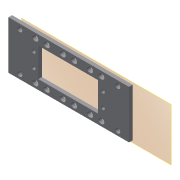
# Autodesk Inventor part: ExtendedServoMount
Saved by Autodesk Inventor 2018 (Build 220112000, 112)
## iProperties
Created: 2018-12-08
Part Number: ExtendedServoMount
Material: Generic
Document SubType Name: Modeling
Designer: ball
Density: 1 g/cm^3
Appearance: Default
Author: ball
Autodesk Inventor part; units mm, degrees
ref_plane "YZ Plane" through (0, 0, 0) normal (1, 0, 0) x (0, 1, 0)
ref_plane "XZ Plane" through (0, 0, 0) normal (0, 1, 0) x (-1, 0, 0)
ref_plane "XY Plane" through (0, 0, 0) normal (0, 0, 1) x (1, 0, 0)
ref_plane "Work Plane1" through (0, 0, 0) normal (0, 0, 1) x (1, 0, 0)
sketch "Sketch2" plane through (0, 0, 0) normal (0, 0, 1) x (1, 0, 0)
  arc A0 (-24.5984, 11.6916) -> (-24.5984, 15.2476) centre (-24.5984, 13.4696) ccw projected
  line L0 (-24.5984, 15.2476) -> (-25.3604, 15.2476) projected
  line L1 (-25.3604, 11.6916) -> (-24.5984, 11.6916) projected
  arc A1 (-25.3604, 15.2476) -> (-25.3604, 11.6916) centre (-25.3604, 13.4696) ccw projected
  arc A2 (-25.3604, 15.2476) -> (-25.3604, 11.6916) centre (-25.3604, 13.4696) ccw
  arc A3 (-24.5984, 11.6916) -> (-24.5984, 15.2476) centre (-24.5984, 13.4696) ccw
  line L2 (-27.1384, 13.4696) -> (-22.8204, 13.4696) construction
  line L3 (-25.3604, 11.6916) -> (-24.5984, 11.6916)
  line L4 (-24.5984, 15.2476) -> (-25.3604, 15.2476)
  arc A4 (-25.3604, 15.2476) -> (-25.3604, 11.6916) centre (-25.3604, 13.4696) ccw
  arc A5 (-24.5984, 11.6916) -> (-24.5984, 15.2476) centre (-24.5984, 13.4696) ccw
  arc A6 (-33.2496, 15.2476) -> (-33.2496, 11.6916) centre (-33.2496, 13.4696) ccw
  arc A7 (-32.4876, 11.6916) -> (-32.4876, 15.2476) centre (-32.4876, 13.4696) ccw
  arc A8 (-43.6499, 11.6916) -> (-43.6499, 15.2476) centre (-43.6499, 13.4696) ccw
  arc A9 (-44.4119, 15.2476) -> (-44.4119, 11.6916) centre (-44.4119, 13.4696) ccw projected
  arc A10 (-51.5391, 11.6916) -> (-51.5391, 15.2476) centre (-51.5391, 13.4696) ccw
  arc A11 (-52.3011, 15.2476) -> (-52.3011, 11.6916) centre (-52.3011, 13.4696) ccw projected
  line L5 (-46.1899, 13.4696) -> (-41.8719, 13.4696) construction
  line L6 (-44.4119, 11.6916) -> (-43.6499, 11.6916)
  line L7 (-43.6499, 15.2476) -> (-44.4119, 15.2476)
  arc A12 (-44.4119, 15.2476) -> (-44.4119, 11.6916) centre (-44.4119, 13.4696) ccw
  arc A13 (-43.6499, 11.6916) -> (-43.6499, 15.2476) centre (-43.6499, 13.4696) ccw
  line L8 (-54.0791, 13.4696) -> (-49.7611, 13.4696) construction
  line L9 (-52.3011, 11.6916) -> (-51.5391, 11.6916)
  line L10 (-51.5391, 15.2476) -> (-52.3011, 15.2476)
  arc A14 (-52.3011, 15.2476) -> (-52.3011, 11.6916) centre (-52.3011, 13.4696) ccw
  arc A15 (-51.5391, 11.6916) -> (-51.5391, 15.2476) centre (-51.5391, 13.4696) ccw
  line L11 (-35.0276, 13.4696) -> (-30.7096, 13.4696) construction
  line L12 (-33.2496, 11.6916) -> (-32.4876, 11.6916)
  line L13 (-32.4876, 15.2476) -> (-33.2496, 15.2476)
  arc A16 (-33.2496, 15.2476) -> (-33.2496, 11.6916) centre (-33.2496, 13.4696) ccw
  arc A17 (-32.4876, 11.6916) -> (-32.4876, 15.2476) centre (-32.4876, 13.4696) ccw
  line L14 (-65.2414, 13.4696) -> (-60.9234, 13.4696) construction
  line L15 (-63.4634, 11.6916) -> (-62.7014, 11.6916)
  line L16 (-62.7014, 15.2476) -> (-63.4634, 15.2476)
  arc A18 (-63.4634, 15.2476) -> (-63.4634, 11.6916) centre (-63.4634, 13.4696) ccw
  arc A19 (-62.7014, 11.6916) -> (-62.7014, 15.2476) centre (-62.7014, 13.4696) ccw
  line L17 (-73.1307, 13.4696) -> (-68.8127, 13.4696) construction
  line L18 (-71.3527, 11.6916) -> (-70.5907, 11.6916)
  line L19 (-70.5907, 15.2476) -> (-71.3527, 15.2476)
  arc A20 (-71.3527, 15.2476) -> (-71.3527, 11.6916) centre (-71.3527, 13.4696) ccw
  arc A21 (-70.5907, 11.6916) -> (-70.5907, 15.2476) centre (-70.5907, 13.4696) ccw
  line L20 (-73.1307, -13.4696) -> (-68.8127, -13.4696) construction
  line L21 (-71.3527, -15.2476) -> (-70.5907, -15.2476)
  line L22 (-70.5907, -11.6916) -> (-71.3527, -11.6916)
  arc A22 (-71.3527, -11.6916) -> (-71.3527, -15.2476) centre (-71.3527, -13.4696) ccw
  arc A23 (-70.5907, -15.2476) -> (-70.5907, -11.6916) centre (-70.5907, -13.4696) ccw
  line L23 (-65.2414, -13.4696) -> (-60.9234, -13.4696) construction
  line L24 (-63.4634, -15.2476) -> (-62.7014, -15.2476)
  line L25 (-62.7014, -11.6916) -> (-63.4634, -11.6916)
  arc A24 (-63.4634, -11.6916) -> (-63.4634, -15.2476) centre (-63.4634, -13.4696) ccw
  arc A25 (-62.7014, -15.2476) -> (-62.7014, -11.6916) centre (-62.7014, -13.4696) ccw
  line L26 (-54.0791, -13.4696) -> (-49.7611, -13.4696) construction
  line L27 (-52.3011, -15.2476) -> (-51.5391, -15.2476)
  line L28 (-51.5391, -11.6916) -> (-52.3011, -11.6916)
  arc A26 (-52.3011, -11.6916) -> (-52.3011, -15.2476) centre (-52.3011, -13.4696) ccw
  arc A27 (-51.5391, -15.2476) -> (-51.5391, -11.6916) centre (-51.5391, -13.4696) ccw
  line L29 (-46.1899, -13.4696) -> (-41.8719, -13.4696) construction
  line L30 (-44.4119, -15.2476) -> (-43.6499, -15.2476)
  line L31 (-43.6499, -11.6916) -> (-44.4119, -11.6916)
  arc A28 (-44.4119, -11.6916) -> (-44.4119, -15.2476) centre (-44.4119, -13.4696) ccw
  arc A29 (-43.6499, -15.2476) -> (-43.6499, -11.6916) centre (-43.6499, -13.4696) ccw
  line L32 (-35.0276, -13.4696) -> (-30.7096, -13.4696) construction
  line L33 (-33.2496, -15.2476) -> (-32.4876, -15.2476)
  line L34 (-32.4876, -11.6916) -> (-33.2496, -11.6916)
  arc A30 (-33.2496, -11.6916) -> (-33.2496, -15.2476) centre (-33.2496, -13.4696) ccw
  arc A31 (-32.4876, -15.2476) -> (-32.4876, -11.6916) centre (-32.4876, -13.4696) ccw
  line L35 (-27.1384, -13.4696) -> (-22.8204, -13.4696) construction
  line L36 (-25.3604, -15.2476) -> (-24.5984, -15.2476)
  line L37 (-24.5984, -11.6916) -> (-25.3604, -11.6916)
  arc A32 (-25.3604, -11.6916) -> (-25.3604, -15.2476) centre (-25.3604, -13.4696) ccw
  arc A33 (-24.5984, -15.2476) -> (-24.5984, -11.6916) centre (-24.5984, -13.4696) ccw
  circle A34 centre (-72.1182, 4.953) radius 1.3525
  circle A35 centre (-72.1182, -4.953) radius 1.3525
  circle A36 centre (-23.8328, -4.953) radius 1.3525
  circle A37 centre (-23.8328, 4.953) radius 1.3525
  line L38 (-68.8127, 10.036) -> (-27.1475, 10.036)
  line L39 (-27.1475, 10.036) -> (-27.1475, -10.16)
  line L40 (-27.1475, -10.16) -> (-68.8127, -10.16)
  line L41 (-68.8127, -10.16) -> (-68.8127, 10.036)
  circle A38 centre (-81.7796, 13.4704) radius 1.778
  circle A39 centre (-81.7796, -13.4704) radius 1.778
  circle A40 centre (-81.7796, 13.4704) radius 1.778
  circle A41 centre (-81.7796, -13.4704) radius 1.778
  circle A42 centre (-13.4704, 13.4704) radius 1.778
  circle A43 centre (-13.4704, -13.4704) radius 1.778
  circle A44 centre (-13.4704, -13.4704) radius 1.778
  circle A45 centre (-13.4704, 13.4704) radius 1.778
  circle A46 centre (-89.6704, 13.4704) radius 1.778
  circle A47 centre (-89.6704, -13.4704) radius 1.778
  circle A48 centre (-5.5796, -13.4704) radius 1.778
  circle A49 centre (-5.5796, 13.4704) radius 1.778
  line L42 (-89.6704, 16.764) -> (-5.5796, 16.764)
  line L43 (-5.5796, 16.764) -> (-5.5796, -16.764)
  line L44 (-5.5796, -16.764) -> (-89.6704, -16.764)
  line L45 (-89.6704, -16.764) -> (-89.6704, 16.764)
  point P0 (0, 0)
  point P1 (-24.9794, 13.4696)
  point P2 (-44.0309, 13.4696)
  point P3 (-51.9201, 13.4696)
  point P4 (-32.8686, 13.4696)
  point P5 (-63.0824, 13.4696)
  point P6 (-70.9717, 13.4696)
  point P7 (-70.9717, -13.4696)
  point P8 (-63.0824, -13.4696)
  point P9 (-51.9201, -13.4696)
  point P10 (-44.0309, -13.4696)
  point P11 (-32.8686, -13.4696)
  point P12 (-24.9794, -13.4696)
  constraints: 112 end point, 92 point on circle, 48 tangent, 46 centre point, 24 point on line, 16 parallel, 12 midpoint, 4 coincident, 4 concentric, 2 horizontal, 2 perpendicular, 40 other
extrude "Extrusion1" add sketch "Sketch2" along normal blind 2.54 contours A46 L45 | A46 L45 L42 L43 A49 A48 L44 A47 | A47 L45 | L43 A49 | L43 A48 picked at (-89.0777, 13.4704) picked at (-89.0777, -13.4704) picked at (-6.7028, 13.6737) picked at (-6.7028, -13.2671)
body "Solid1"
